# Autodesk Inventor part: SPINN2_V2
Saved by Autodesk Inventor 2015 SP1 (Build 190203100, 203)
## iProperties
Created: 2015-06-25
Part Number: SPINN2_V2
Material: Generic
Document SubType Name: Modeling
Designer: Patrick
Density: 1 g/cm^3
Appearance: 300BGA, SPINN2_V2
Author: Patrick
Autodesk Inventor part; units mm, degrees
ref_plane "YZ Plane" through (0, 0, 0) normal (1, 0, 0) x (0, 1, 0)
ref_plane "XZ Plane" through (0, 0, 0) normal (0, 1, 0) x (-1, 0, 0)
ref_plane "XY Plane" through (0, 0, 0) normal (0, 0, 1) x (1, 0, 0)
sketch "300BGA, SPINN2_V2_71" plane through (0, 0, 0) normal (0, 0, 1) x (1, 0, 0)
  line L0 (-9.625, -9.625) -> (-9.625, 9.625)
  line L1 (-9.625, 9.625) -> (9.725, 9.625)
  line L2 (9.725, 9.625) -> (9.725, -9.625)
  line L3 (9.725, -9.625) -> (-9.625, -9.625)
  constraints: 8 end point
extrude "Extrusion1" add sketch "300BGA, SPINN2_V2_71" along normal blind 1
body "Solid1"
